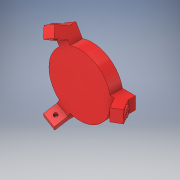
# Autodesk Inventor part: BottomPlatform
Saved by Autodesk Inventor 2019 (Build 230136000, 136)
## iProperties
Created: 2022-07-06
Part Number: BottomPlatform
Material: Generic
Document SubType Name: Modeling
Designer: zreik
Density: 1 g/cm^3
Appearance: Light Red
Author: zreik
Autodesk Inventor part; units mm, degrees
ref_plane "YZ Plane" through (0, 0, 0) normal (1, 0, 0) x (0, 1, 0)
ref_plane "XZ Plane" through (0, 0, 0) normal (0, 1, 0) x (-1, 0, 0)
ref_plane "XY Plane" through (0, 0, 0) normal (0, 0, 1) x (1, 0, 0)
sketch "Sketch1" plane through (0, 0, 0) normal (0, 0, 1) x (1, 0, 0)
  circle A0 centre (0, 0) radius 25
  line L0 (15, -5) -> (35, -5)
  line L1 (35, -5) -> (35, 5)
  line L2 (35, 5) -> (15, 5)
  line L3 (15, 5) -> (15, -5)
  line L4 (15, -5) -> (35, 5) construction
  line L5 (35, -5) -> (15, 5) construction
  point P0 (25, 0)
  dimension "d0" = 50
  dimension "d3" = 10
  dimension "d4" = 20
  dimension "d5" = 0
  constraints: 12 end point, 2 midpoint, 2 parallel, 1 coincident, 1 horizontal, 1 horizontal alignment, 1 perpendicular, 2 other
  measures "d3" distance of L0.end L1.end
  measures "d4" distance of L0.start L0.end
  measures "d5" vertical distance of point (0, 0) point (25, 0)
extrude "Extrusion1" add sketch "Sketch1" along normal mid plane 10 contours A0 L0 L3 L2 | L2 L3 L0 A0
extrude "Extrusion2" add sketch "Sketch1" along normal mid plane 10 contours A0 L0 L3 L2 | A0 L2 L1 L0 picked at (18.3333, 0)
chamfer "Chamfer1" distance 7 angle 30 1 edges at (35, 0, 5) measured on face at (34.5, 0, 5)
sketch "Sketch2" plane through (28, -5, 5) normal (0.5, 0, 0.8660254) x (0.8660254, 0, -0.5)
  line L0 (8.0829, 0) -> (0, 0)
  line L1 (0, 0) -> (0, 10)
  line L2 (0, 10) -> (8.0829, 10)
  line L3 (8.0829, 10) -> (8.0829, 0)
  line L4 (8.0829, 0) -> (0, 10) construction
  line L5 (0, 0) -> (8.0829, 10) construction
  line L6 (0, 10) -> (0, 0) projected
  line L7 (8.0829, 0) -> (8.0829, 10) projected
  line L8 (8.0829, 10) -> (0, 10) projected
  line L9 (0, 0) -> (8.0829, 0) projected
  point P0 (-21.7487, 5)
  point P1 (4.0415, 5)
  dimension "d11" = 0
  dimension "d12" = 0
  dimension "d13" = 0
  dimension "d14" = 0
  constraints: 12 end point, 2 midpoint, 2 parallel, 1 horizontal, 1 perpendicular
  measures "d11" distance between parallel lines of L1 L6
  measures "d12" distance between parallel lines of L7 L3
  measures "d13" distance between parallel lines of L8 L2
  measures "d14" distance between parallel lines of L9 L0
extrude "Extrusion3" add sketch "Sketch2" along normal blind 10
sketch "Sketch3" plane through (28, -5, 5) normal (-0.8660254, 0, 0.5) x (0.5, 0, 0.8660254)
  circle A0 centre (5, 5) radius 1.5
  line L0 (10, 10) -> (10, 0) projected
  line L1 (0, 10) -> (0, 0) projected
  line L2 (0, 0) -> (10, 0) projected
  line L3 (0, 10) -> (10, 10) projected
  point P0 (-18.3301, 5)
  dimension "d17" = 3
  dimension "d18" = 5
  dimension "d19" = 5
  dimension "d20" = 5
  dimension "d21" = 5
  constraints: 1 centre point
  measures "d17" diameter of A0
  measures "d18" distance from line of L0 A0.centre
  measures "d19" distance from line of L1 A0.centre
  measures "d20" distance from line of L2 A0.centre
  measures "d21" distance from line of L3 A0.centre
extrude "Extrusion8" cut sketch "Sketch3" against normal through all contours A0
sketch "Sketch6" plane through (35, -5, 0.9585) normal (0.8660254, 0, -0.5) x (-0.5, 0, -0.8660254)
  circle A0 centre (-5, 5) radius 3.5
  circle A1 centre (-5, 5) radius 1.5 projected
  point P0 (18.3301, 5)
  dimension "d40" = 7
  constraints: 1 centre point, 1 concentric
  measures "d40" diameter of A0
extrude "Extrusion9" add sketch "Sketch6" along normal blind 1
chamfer "Chamfer3" distance 1 angle 45 1 edges at (39.25, 0, 8.3198)
pattern_circular "Circular Pattern1" count 3 over 360 about axis through (0, 0, 0) along (0, 0, 1) of "Extrusion3", "Extrusion2", "Chamfer1", "Extrusion8", "Chamfer3", "Extrusion9"
equation "\"d18\" = d19"
equation "\"d20\" = d21"
body "Solid1"
